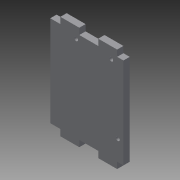
# Autodesk Inventor part: arduino-fix
Saved by Autodesk Inventor 2014 (Build 180170000, 170)
## iProperties
Created: 2014-03-02
Part Number: arduino-fix
Material: 常规
Document SubType Name: Modeling
Designer: Keshuai
Density: 1 g/cm^3
Appearance: 默认
Author: Keshuai
Autodesk Inventor part; units mm, degrees
ref_plane "YZ Plane" through (0, 0, 0) normal (1, 0, 0) x (0, 1, 0)
ref_plane "XZ Plane" through (0, 0, 0) normal (0, 1, 0) x (-1, 0, 0)
ref_plane "XY Plane" through (0, 0, 0) normal (0, 0, 1) x (1, 0, 0)
sketch "草图2" plane through (0, 0, 0) normal (0, 1, 0) x (-1, 0, 0)
  line L0 (2, 0) -> (-13, 0) projected
  line L1 (2, 0) -> (2, -5) projected
  line L2 (-13, -5) -> (2, -5) projected
  line L3 (-13, 0) -> (-13, -5) projected
  line L4 (-28, 0) -> (-43, 0) projected
  line L5 (-28, 0) -> (-28, -5) projected
  line L6 (-43, -5) -> (-28, -5) projected
  line L7 (-43, 0) -> (-43, -5) projected
  line L8 (-48, 0) -> (-48, -5) projected
  line L9 (15, 0) -> (15, -5) projected
  line L10 (23, 72) -> (15, 72) projected
  line L11 (-48, 0) -> (10, 0)
  line L12 (10, 0) -> (10, 72)
  line L13 (10, 72) -> (-48, 72)
  line L14 (-48, 72) -> (-48, 0)
  line L15 (7.3, 2) -> (-46, 2) construction
  line L16 (-46, 2) -> (-46, 70.6) construction
  line L17 (-46, 70.6) -> (7.3, 70.6) construction
  line L18 (7.3, 70.6) -> (7.3, 2) construction
  circle A0 centre (-43.5, 16) radius 1.5
  circle A1 centre (-38.4, 68.1) radius 1.5
  circle A2 centre (-10.5, 68.1) radius 1.5
  line L19 (2, 72) -> (-13, 72)
  line L20 (-13, 72) -> (-13, 77)
  line L21 (-13, 77) -> (2, 77)
  line L22 (2, 77) -> (2, 72)
  line L23 (-28, 72) -> (-43, 72)
  line L24 (-43, 72) -> (-43, 77)
  line L25 (-43, 77) -> (-28, 77)
  line L26 (-28, 77) -> (-28, 72)
  point P0 (0, 0)
  dimension "d1" = 53.3
  dimension "d2" = 68.6
  dimension "d3" = 2
  dimension "d4" = 2
  dimension "d5" = 5
  dimension "d6" = 3
  dimension "d7" = 14
  dimension "d8" = 2.5
  dimension "d9" = 3
  dimension "d10" = 5.1
  dimension "d11" = 52.1
  dimension "d12" = 3
  dimension "d13" = 27.9
  dimension "d14" = 5
  constraints: 32 end point, 8 parallel, 4 horizontal, 4 perpendicular, 3 centre point, 2 point on line
  measures "d1" distance of L16.end L17.end
  measures "d2" distance of L15.end L16.end
  measures "d3" distance between parallel lines of L11 L15
  measures "d4" distance between parallel lines of L14 L16
  measures "d5" distance from line of L10.end L12
  measures "d6" diameter of A0
  measures "d7" distance from line of L15 A0.centre
  measures "d8" distance from line of L16 A0.centre
  measures "d9" diameter of A1
  measures "d10" horizontal distance of A0.centre A1.centre
  measures "d11" vertical distance of A0.centre A1.centre
  measures "d12" diameter of A2
  measures "d13" distance of A1.centre A2.centre
  measures "d14" distance of L19.end L20.end
extrude "拉伸1" add sketch "草图2" along normal blind 5
